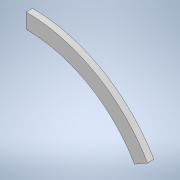
# Autodesk Inventor part: SideB
Saved by Autodesk Inventor 2021.1 (Build 251245010, 245A)
## iProperties
Created: 2020-10-17
Part Number: SideB
Material: Generic
Document SubType Name: Modeling
Designer: robst
Density: 1 g/cm^3
Appearance: Default
Author: robst
Autodesk Inventor part; units mm, degrees
ref_plane "YZ Plane" through (0, 0, 0) normal (1, 0, 0) x (0, 1, 0)
ref_plane "XZ Plane" through (0, 0, 0) normal (0, 1, 0) x (-1, 0, 0)
ref_plane "XY Plane" through (0, 0, 0) normal (0, 0, 1) x (1, 0, 0)
sketch "Sketch1" plane through (0, 0, 0) normal (0, 0, 1) x (1, 0, 0)
  arc A0 (439.9409, 254) -> (0, 508) centre (0, 0) ccw
  arc A1 (432.2419, 249.555) -> (0, 499.11) centre (0, 0) ccw
  arc A2 (483.935, 279.4) -> (0, 558.8) centre (0, 0) ccw
  line L0 (0, 0) -> (0, 558.8)
  line L1 (0, 0) -> (483.935, 279.4)
  dimension "d0" = 1016
  dimension "d1" = 8.89
  dimension "d2" = 50.8
  dimension "d3" = 60
  constraints: 6 point on circle, 4 end point, 4 point on line, 3 centre point, 3 coincident, 1 vertical
  measures "d0" diameter of A0
  measures "d1" radial gap between concentric circles of A1 A0
  measures "d2" radial gap between concentric circles of A2 A0
  measures "d3" angle of L1 L0
extrude "Extrusion1" add sketch "Sketch1" against normal blind 25.4 contours L1 A1 L0 A0 | A0 L0 A2 L1
body "Solid1"
